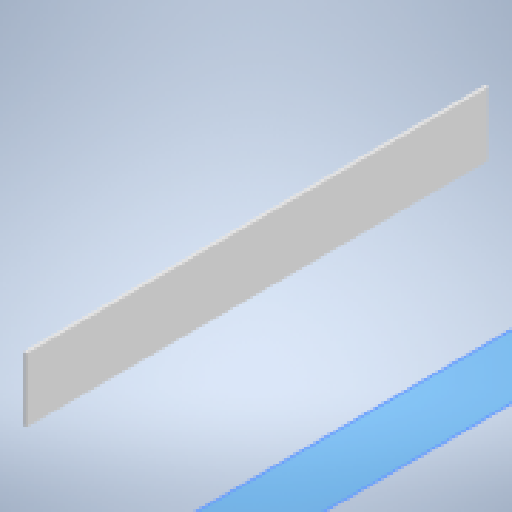
# Autodesk Inventor part: TableroVertical2
Saved by Autodesk Inventor 2024 (Build 280153000, 153)
## iProperties
Created: 2023-07-03
Part Number: TableroVertical2
Material: Genérico
Document SubType Name: Modeling
Designer: sergi
Density: 1 g/cm^3
Appearance: Valor por defecto
Author: sergi
Autodesk Inventor part; units mm, degrees
ref_plane "YZ Plane" through (0, 0, 0) normal (1, 0, 0) x (0, 1, 0)
ref_plane "XZ Plane" through (0, 0, 0) normal (0, 1, 0) x (-1, 0, 0)
ref_plane "XY Plane" through (0, 0, 0) normal (0, 0, 1) x (1, 0, 0)
sketch "Boceto1" plane through (0, 0, 0) normal (0, 1, 0) x (-1, 0, 0)
  line L0 (0, 0) -> (-16, 0)
  line L1 (-16, 0) -> (-16, -2172)
  line L2 (-16, -2172) -> (0, -2172)
  line L3 (0, -2172) -> (0, 0)
  line L4 (1484, -1375) -> (-16, -1375) projected
  line L5 (-16, -1375) -> (-16, -1972) projected
  line L6 (-16, -1972) -> (1484, -1972) projected
  line L7 (1484, -1972) -> (1484, -1375) projected
  line L8 (-16, -1972) -> (0, -1972)
  line L9 (1459, -1956) -> (-16, -1956) projected
  point P0 (0, -1956)
  dimension "d0" = 16
  dimension "d1" = 2172
  constraints: 10 end point, 2 parallel, 2 point on line, 1 horizontal, 1 perpendicular
  measures "d0" distance of L2.end L1.end
  measures "d1" distance of L1.end L0.end
extrude "Extrusión1" add sketch "Boceto1" along normal blind 300 contours L3 L4 L1 L0 | L3 L9 L1 L4
